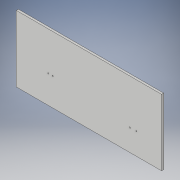
# Autodesk Inventor part: PossibleTopPlate
Saved by Autodesk Inventor 2017 (Build 210142000, 142)
## iProperties
Created: 2017-12-09
Part Number: PossibleTopPlate
Material: Generic
Document SubType Name: Modeling
Designer: User
Density: 1 g/cm^3
Appearance: Default
Author: User
Autodesk Inventor part; units mm, degrees
ref_plane "YZ Plane" through (0, 0, 0) normal (1, 0, 0) x (0, 1, 0)
ref_plane "XZ Plane" through (0, 0, 0) normal (0, 1, 0) x (-1, 0, 0)
ref_plane "XY Plane" through (0, 0, 0) normal (0, 0, 1) x (1, 0, 0)
sketch "Sketch1" plane through (0, 0, 0) normal (0, 0, 1) x (1, 0, 0)
  line L0 (0, 0) -> (431.8, 0)
  line L1 (431.8, 0) -> (431.8, 152.4)
  line L2 (431.8, 152.4) -> (0, 152.4)
  line L3 (0, 152.4) -> (0, 0)
  dimension "d0" = 431.8
  dimension "d1" = 152.4
  constraints: 8 end point, 2 parallel, 1 horizontal, 1 perpendicular
  measures "d0" distance of L2.end L1.end
  measures "d1" distance of L1.end L0.end
extrude "Extrusion1" add sketch "Sketch1" along normal blind 6.35
thicken "Thicken1" operation add thickness 44.45 both sides no extend neighbours yes toward (0, 1, 0) faces at (287.8667, 152.4, 4.2333)
sketch "Sketch3" plane through (0, 0, 0) normal (0, 0, -1) x (-1, 0, 0)
  line L0 (0, 196.85) -> (0, 0) projected
  line L1 (0, 0) -> (-431.8, 0) projected
  line L2 (-88.9, 0) -> (-88.9, 77.724)
  line L3 (-88.9, 0) -> (-11.176, 0) construction
  line L4 (-88.9, 77.724) -> (0, 77.724)
  line L5 (0, 196.85) -> (0, 0) projected
  line L6 (-88.9, 77.724) -> (-114.3, 77.724)
  line L7 (-114.3, 77.724) -> (-114.3, 87.249)
  line L8 (-114.3, 87.249) -> (-88.9, 87.249)
  line L9 (-88.9, 87.249) -> (-88.9, 77.724)
  line L10 (-88.9, 82.4865) -> (-95.25, 82.4865)
  line L11 (-114.3, 82.4865) -> (-107.95, 82.4865)
  dimension "d8" = 77.724
  dimension "d9" = 90
  dimension "d10" = 88.9
  dimension "d11" = 25.4
  dimension "d12" = 9.525
  dimension "d13" = 6.35
  dimension "d14" = 6.35
  constraints: 18 end point, 5 horizontal, 3 perpendicular, 2 coincident, 2 midpoint, 2 parallel, 2 point on line
  measures "d8" distance of L2.start L2.end
  measures "d9" angle of L3 L2
  measures "d10" distance of L4.end L2.end
  measures "d11" distance of L7.end L8.end
  measures "d12" distance of L6.end L7.end
  measures "d13" distance of L10.start L10.end
  measures "d14" distance of L11.start L11.end
hole "Hole1" at (107.95, 82.4865, 0) at (95.25, 82.4865, 0) direction (0, 0, 1) diameter 3.302 depth 25.4 tip angle 118
sketch "Sketch5" plane through (0, 0, 0) normal (0, 0, -1) x (-1, 0, 0)
  line L0 (-431.8, 0) -> (-431.8, 196.85) projected
  line L1 (-431.8, 59.69) -> (-369.57, 59.69)
  line L2 (-431.8, 59.69) -> (-369.57, 59.69) construction
  line L3 (0, 0) -> (-431.8, 0) projected
  line L4 (-369.57, 0) -> (-369.57, 59.69)
  line L5 (-369.57, 0) -> (-309.88, 0) construction
  line L6 (-369.57, 59.69) -> (-325.12, 59.69)
  line L7 (-325.12, 59.69) -> (-325.12, 69.215)
  line L8 (-325.12, 69.215) -> (-369.57, 69.215)
  line L9 (-369.57, 69.215) -> (-369.57, 59.69)
  line L10 (-369.57, 64.4525) -> (-356.87, 64.4525)
  line L11 (-325.12, 64.4525) -> (-337.82, 64.4525)
  dimension "d22" = 62.23
  dimension "d23" = 0
  dimension "d24" = 59.69
  dimension "d25" = 90
  dimension "d26" = 0
  dimension "d27" = 44.45
  dimension "d28" = 9.525
  dimension "d29" = 12.7
  dimension "d30" = 12.7
  constraints: 20 end point, 5 horizontal, 3 perpendicular, 2 coincident, 2 equal length, 2 midpoint, 2 parallel, 2 point on line
  measures "d22" distance of L1.start L1.end
  measures "d23" distance between parallel lines of L1 L2
  measures "d24" distance of L4.start L4.end
  measures "d25" angle of L5 L4
  measures "d26" distance of L2.end L4.end
  measures "d27" distance of L8.end L7.end
  measures "d28" distance of L7.end L6.end
  measures "d29" distance of L10.start L10.end
  measures "d30" distance of L11.start L11.end
hole "Hole2" at (356.87, 64.4525, 0) at (337.82, 64.4525, 0) direction (0, 0, 1) diameter 3.302 depth 25.4 tip angle 118
body "Solid1"
